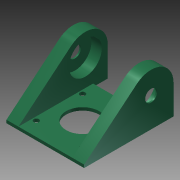
# Autodesk Inventor part: Worm Gear Box
Saved by Autodesk Inventor 2015 SP1 (Build 190203100, 203)
## iProperties
Created: 2015-03-03
Part Number: Worm Gear Box
Material: PC/ABS Plastic
Document SubType Name: Modeling
Designer: Andrew
Density: 0.357273 g/cm^3
Appearance: Smooth - Dark Sea Green
Author: Andrew
Autodesk Inventor part; units mm, degrees
ref_plane "YZ Plane" through (0, 0, 0) normal (1, 0, 0) x (0, 1, 0)
ref_plane "XZ Plane" through (0, 0, 0) normal (0, 1, 0) x (-1, 0, 0)
ref_plane "XY Plane" through (0, 0, 0) normal (0, 0, 1) x (1, 0, 0)
sketch "Sketch1" plane through (0, 0, 0) normal (0, 0, 1) x (1, 0, 0)
  circle A0 centre (-15.5, 15.5) radius 1.75
  circle A1 centre (15.5, 15.5) radius 1.75
  circle A2 centre (-15.5, -15.5) radius 1.75
  circle A3 centre (15.5, -15.5) radius 1.75
  circle A4 centre (0, 0) radius 11.05
  line L0 (-15.5, 15.5) -> (15.5, 15.5) construction
  line L1 (15.5, 15.5) -> (15.5, -15.5) construction
  line L2 (15.5, -15.5) -> (-15.5, -15.5) construction
  line L3 (-15.5, -15.5) -> (-15.5, 15.5) construction
  line L4 (-15.5, 15.5) -> (15.5, -15.5) construction
  line L5 (15.5, 15.5) -> (-15.5, -15.5) construction
  line L6 (-25, 25) -> (-25, -25)
  line L7 (-25, -25) -> (25, -25)
  line L8 (25, -25) -> (25, 25)
  line L9 (25, 25) -> (-25, 25)
  dimension "d0" = 22.1
  dimension "d1" = 31
  dimension "d2" = 31
  dimension "d3" = 3.5
  dimension "d4" = 50
  dimension "d5" = 50
  constraints: 20 end point, 6 perpendicular, 5 centre point, 3 equal radius, 2 coincident, 2 point on line, 1 horizontal, 1 midpoint, 1 vertical
  measures "d0" diameter of A4
  measures "d1" distance of L2.end L0.start
  measures "d2" distance of L0.end L0.start
  measures "d3" diameter of A1
  measures "d4" distance of L7.end L8.end
  measures "d5" distance of L6.end L7.end
extrude "Extrusion1" add sketch "Sketch1" against normal blind 2
sketch "Sketch2" plane through (25, -25, 0) normal (1, 0, 0) x (0, 0, -1)
  line L0 (0, 0) -> (0, 50) projected
  line L1 (0, 0) -> (2, 0) projected
  line L2 (2, 50) -> (2, 0) projected
  line L3 (0, 50) -> (2, 50) projected
  line L4 (0, 0) -> (0, 50) projected
  line L5 (0, 59.85) -> (-17.583, 59.85)
  line L6 (-29.1492, 35.2989) -> (0, 0)
  line L7 (0, 38.75) -> (0, 42.25) construction
  line L8 (0, 44.85) -> (-34.6915, 44.85) construction
  line L9 (2, 50) -> (2, 59.85)
  line L10 (2, 59.85) -> (0, 59.85)
  circle A0 centre (-17.583, 44.85) radius 4
  circle A1 centre (-17.583, 44.85) radius 11
  circle A2 centre (-17.583, 44.85) radius 13
  arc A3 (-17.583, 59.85) -> (-29.1492, 35.2989) centre (-17.583, 44.85) ccw
  point P0 (0, 25)
  dimension "d8" = 19.85
  dimension "d9" = 19.583
  dimension "d10" = 8
  dimension "d11" = 22
  dimension "d12" = 2
  dimension "d13" = 2
  constraints: 10 end point, 4 centre point, 4 coincident, 3 perpendicular, 3 point on line, 2 point on circle, 2 tangent, 1 vertical
  measures "d8" distance from line of point (0, 25) L8
  measures "d9" distance from line of L2 point (-17.583, 44.85)
  measures "d10" diameter of A0
  measures "d11" diameter of A1
  measures "d12" radial gap between concentric circles of A1 A2
  measures "d13" radial gap between concentric circles of A2 A3
extrude "Extrusion2" add sketch "Sketch2" against normal blind 7 contours L6 A3 L5 L10 L9 L3 L0 | A2
extrude "Extrusion3" add sketch "Sketch2" along normal blind 1 contours L6 A3 L5 L10 L9 L3 L0 | L0 L3 L2 L1 | A1 | A2
mirror "Mirror1" about plane through (0, 0, 0) normal (1, 0, 0) of "Extrusion2", "Extrusion3"
body "Solid1"
